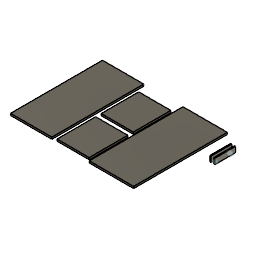
folding (Autodesk Fusion 360 design; units mm, degrees)
Autodesk Fusion 360 part; units mm, degrees
sketch "Sketch1" plane through (0, 0, 0) normal (0, 0, 1) x (1, 0, 0)
  line L0 (-100, 50) -> (-55.6348, 50)
  line L1 (-55.6348, 50) -> (-55.6348, -48.6805)
  line L2 (-55.6348, -48.6805) -> (-100, -48.6805)
  line L3 (-100, -48.6805) -> (-100, 50)
  line L4 (-13.698, 50) -> (33.9288, 50)
  line L5 (33.9288, 50) -> (33.9288, -50.5771)
  line L6 (33.9288, -50.5771) -> (-13.698, -50.5771)
  line L7 (-13.698, -50.5771) -> (-13.698, 50)
  line L8 (-51.2094, 40.0402) -> (-16.6483, 40.0402)
  line L9 (-16.6483, 40.0402) -> (-16.6483, -0.2886)
  line L10 (-16.6483, -0.2886) -> (-51.2094, -0.2886)
  line L11 (-51.2094, -0.2886) -> (-51.2094, 40.0402)
  line L12 (-51.2094, -6.1114) -> (-16.6483, -6.1114)
  line L13 (-16.6483, -6.1114) -> (-16.6483, -47.6268)
  line L14 (-16.6483, -47.6268) -> (-51.2094, -47.6268)
  line L15 (-51.2094, -47.6268) -> (-51.2094, -6.1114)
extrude "BaseFlange1" add sketch "Sketch1" sketch "Sketch1" sketch "Sketch1" sketch "Sketch1" along normal blind 2 contours L4 L5 L6 L7 of sketch 2 contours L4 L5 L6 L7 | L12 L13 L14 L15 of sketch 3 contours L0 L1 L2 L3 | L4 L5 L6 L7 | L12 L13 L14 L15 of sketch 4 makes body 1 at (-39.689, -19.9499, 0) makes body 2 at (-85.2116, -15.787, 0) makes body 3 at (2.1776, -17.0514, 0) makes body 4 at (-28.1687, 13.1544, 0)
sketch "Sketch2" plane through (0, 0, 0) normal (0, 0, 1) x (1, 0, 0)
  line L0 (49.9449, 37.5114) -> (51.2094, 37.5114)
  line L1 (51.2094, 37.5114) -> (51.2094, 15.1731)
  line L2 (51.2094, 15.1731) -> (49.9449, 15.1731)
  line L3 (49.9449, 15.1731) -> (49.9449, 37.5114)
  line L4 (54.0932, 37.5114) -> (55.2761, 37.5114)
  line L5 (55.2761, 37.5114) -> (55.2761, 15.1731)
  line L6 (55.2761, 15.1731) -> (54.0932, 15.1731)
  line L7 (54.0932, 15.1731) -> (54.0932, 37.5114)
  circle A0 centre (52.7272, 34.8211) radius 1.4132
  circle A1 centre (52.7272, 18.7079) radius 1.4399
extrude "Extrude1" add sketch "Sketch2" along normal blind 6 separate body contours L0 L1 L2 L3 | L4 L5 L6 L7 A0 A1 makes body 5 at (51.2094, 30.0653, 2) makes body 6 at (55.2761, 30.0653, 2)
sketch "Sketch3" plane through (0, 0, 0) normal (0, 0, 1) x (1, 0, 0)
  circle A0 centre (52.6844, 34.0307) radius 1.4414
  circle A1 centre (52.6844, 17.8423) radius 1.5272
  point P0 (52.6844, 34.0307)
named bodies: "down -plate", "left-plate", "right-plate", "up-plate"
